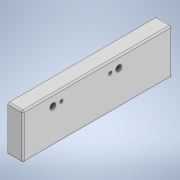
# Autodesk Inventor part: Backplate
Saved by Autodesk Inventor 2022 (Build 260153000, 153)
## iProperties
Created: 2022-03-29
Part Number: Backplate
Material: Generic
Document SubType Name: Modeling
Designer: thoms
Density: 1 g/cm^3
Appearance: Default
Author: thoms
Autodesk Inventor part; units mm, degrees
ref_plane "YZ Plane" through (0, 0, 0) normal (1, 0, 0) x (0, 1, 0)
ref_plane "XZ Plane" through (0, 0, 0) normal (0, 1, 0) x (-1, 0, 0)
ref_plane "XY Plane" through (0, 0, 0) normal (0, 0, 1) x (1, 0, 0)
sketch "Sketch1" plane through (0, 0, 0) normal (1, 0, 0) x (0, 1, 0)
  line L0 (7.5, 25) -> (-7.5, 25)
  line L1 (-7.5, 25) -> (-7.5, -25)
  line L2 (-7.5, -25) -> (7.5, -25)
  line L3 (7.5, -25) -> (7.5, 25)
  point P0 (0, 0)
  dimension "d0" = 50
  dimension "d1" = 25
  dimension "d2" = 15
  dimension "d3" = 7.5
  constraints: 8 end point, 2 parallel, 1 horizontal, 1 perpendicular
  measures "d0" distance of L2.end L0.start
  measures "d1" distance from line of point (0, 0) L0
  measures "d2" distance of L0.start L0.end
  measures "d3" distance from line of point (0, 0) L3
extrude "Extrusion1" add sketch "Sketch1" against normal blind 5
sketch "Sketch2" plane through (0, 0, 0) normal (1, 0, 0) x (0, 0, -1)
  circle A0 centre (-12.1, 4) radius 0.55
  circle A1 centre (-14.95, 4) radius 1
  circle A2 centre (4.25, 4) radius 0.55
  circle A3 centre (7.1, 4) radius 1
  line L0 (25, -7.5) -> (25, 7.5) projected
  line L1 (-25, 7.5) -> (-25, -7.5) projected
  line L2 (-14.95, 4) -> (7.1, 4) construction
  line L3 (-25, -7.5) -> (25, -7.5) projected
  point P0 (0, 0)
  dimension "d6" = 2
  dimension "d7" = 2
  dimension "d8" = 1.1
  dimension "d9" = 1.1
  dimension "d11" = 2.85
  dimension "d13" = 2.85
  dimension "d14" = 10.05
  dimension "d15" = 11.5
  dimension "d19" = 16.35
  constraints: 4 centre point, 2 end point, 1 horizontal
  measures "d6" diameter of A1
  measures "d7" diameter of A3
  measures "d8" diameter of A0
  measures "d9" diameter of A2
  measures "d11" distance of A0.centre L2.start
  measures "d13" distance of L2.end A2.centre
  measures "d14" distance from line of L1 L2.start
  measures "d15" distance between parallel lines of L3 L2
  measures "d19" distance of A2.centre A0.centre
extrude "Extrusion2" cut sketch "Sketch2" against normal up to surface (5 mm away)
fillet "Fillet1" radius 0.5 8 edges at (0, 0, 25) (0, 7.5, 0) (0, 0, -25) (0, -7.5, 0) (-2.5, 7.5, 25) (-2.5, -7.5, 25) (-2.5, 7.5, -25) (-2.5, -7.5, -25)
body "Solid1"
